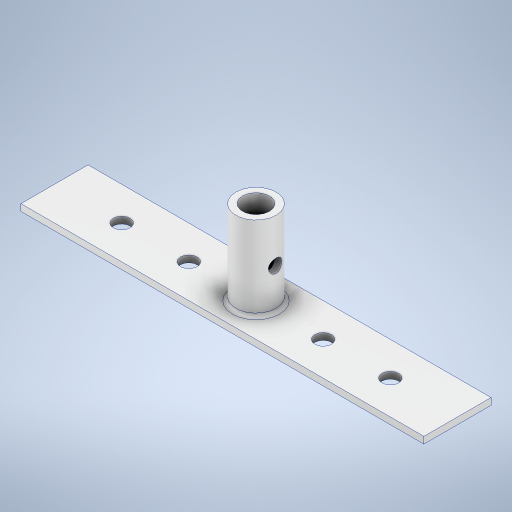
# Autodesk Inventor part: 2020_ax_connector
Saved by Autodesk Inventor 2024 (Build 280153000, 153)
## iProperties
Created: 2025-12-24
Part Number: 2020_ax_connector
Material: Aluminum 6061
Document SubType Name: Modeling
Designer: schar
Density: 2.7 g/cm^3
Appearance: Aluminum - Flat
Author: schar
Autodesk Inventor part; units mm, degrees
ref_plane "YZ Plane" through (0, 0, 0) normal (1, 0, 0) x (0, 1, 0)
ref_plane "XZ Plane" through (0, 0, 0) normal (0, 1, 0) x (-1, 0, 0)
sketch "Sketch1" plane through (0, 0, 0) normal (0, 1, 0) x (-1, 0, 0)
  line L0 (60, 10) -> (-60, 10)
  line L1 (-60, 10) -> (-60, -10)
  line L2 (-60, -10) -> (60, -10)
  line L3 (60, -10) -> (60, 10)
  line L4 (60, 10) -> (-60, -10) construction
  line L5 (-60, 10) -> (60, -10) construction
  line L6 (0, 0) -> (20, 0)
  line L7 (20, 0) -> (40, 0)
  line L8 (0, 0) -> (-20, 0)
  line L9 (-20, 0) -> (-40, 0)
  circle A0 centre (-20, 0) radius 2.5
  circle A1 centre (-40, 0) radius 2.5
  circle A2 centre (20, 0) radius 2.5
  circle A3 centre (40, 0) radius 2.5
  dimension "d0" = 120
  dimension "d1" = 20
  dimension "d2" = 20
  dimension "d3" = 20
  dimension "d4" = 20
  dimension "d5" = 20
  dimension "d6" = 5
  dimension "d7" = 5
  dimension "d8" = 5
  dimension "d9" = 5
  constraints: 20 end point, 4 centre point, 4 coincident, 3 horizontal, 2 midpoint, 2 parallel, 2 point on line, 1 perpendicular
  measures "d0" distance of L2.end L1.end
  measures "d1" distance of L1.end L0.end
  measures "d2" distance of L6.start L6.end
  measures "d3" distance of L6.end L7.end
  measures "d4" distance of L6.start L8.end
  measures "d5" distance of L8.end L9.end
  measures "d6" diameter of A0
  measures "d7" diameter of A1
  measures "d8" diameter of A2
  measures "d9" diameter of A3
extrude "Extrusion1" add sketch "Sketch1" along normal blind 2
sketch "Sketch2" plane through (0, 2, 0) normal (0, 1, 0) x (1, 0, 0)
  circle A0 centre (0, 0) radius 4
  circle A1 centre (0, 0) radius 6
  dimension "d12" = 8
  dimension "d13" = 12
  constraints: 2 centre point, 2 coincident
  measures "d12" diameter of A0
  measures "d13" diameter of A1
extrude "Extrusion2" add sketch "Sketch2" along normal blind 25
fillet "Fillet1" radius 1 1 edges at (-6, 2, 0)
ref_plane "Work Plane1" through (6, 2, 0) normal (1, 0, 0) x (0, 0, -1)
sketch "Sketch3" plane through (6, 2, 0) normal (1, 0, 0) x (0, 0, -1)
  line L0 (0, 0) -> (0, 12)
  circle A0 centre (0, 12) radius 2
  point P0 (0, -2)
  dimension "d17" = 12
  dimension "d18" = 4
  constraints: 2 end point, 1 centre point, 1 coincident, 1 vertical
  measures "d17" distance of L0.start L0.end
  measures "d18" diameter of A0
extrude "Extrusion3" cut sketch "Sketch3" against normal blind 5
thread "Thread1" size "M4x0.7" class "6H" standard "ANSI Metric M Profile" length 15
body "Solid1"
